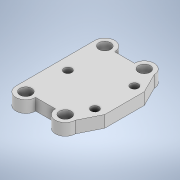
# Autodesk Inventor part: Camera_Mount_DFK33GP006
Saved by Autodesk Inventor 2021 (Build 250183000, 183)
## iProperties
Created: 2022-02-02
Part Number: Camera_Mount_DFK33GP006
Material: Generic
Document SubType Name: Modeling
Designer: Jorian Brusind
Density: 1 g/cm^3
Appearance: Default
Author: Jorian Brusind
Autodesk Inventor part; units mm, degrees
ref_plane "YZ Plane" through (0, 0, 0) normal (1, 0, 0) x (0, 1, 0)
ref_plane "XZ Plane" through (0, 0, 0) normal (0, 1, 0) x (-1, 0, 0)
ref_plane "XY Plane" through (0, 0, 0) normal (0, 0, 1) x (1, 0, 0)
sketch "Sketch1" plane through (0, 0, 0) normal (0, 1, 0) x (-1, 0, 0)
  line L0 (0, 0) -> (40, 0)
  line L1 (40, 0) -> (40, -50)
  line L2 (40, -50) -> (0, -50)
  line L3 (0, -50) -> (0, 0)
  line L4 (0, -25) -> (5, -25)
  line L5 (5, -25) -> (28.7, -25)
  line L6 (5, -25) -> (5, -15)
  line L7 (5, -25) -> (5, -35)
  circle A0 centre (5, -15) radius 2
  circle A1 centre (5, -35) radius 2
  circle A2 centre (28.7, -25) radius 2
  line L8 (40, 0) -> (30, 0)
  line L9 (30, 0) -> (30, -5)
  circle A3 centre (30, -5) radius 3
  circle A4 centre (30, -45) radius 3
  circle A5 centre (10, -5) radius 3
  circle A6 centre (10, -45) radius 3
  circle A7 centre (30, -5) radius 5
  circle A8 centre (10, -5) radius 5
  circle A9 centre (30, -45) radius 5
  circle A10 centre (10, -45) radius 5
  line L10 (0, -15) -> (5, -15)
  line L11 (5, -35) -> (0, -35)
  line L12 (10, -5) -> (5, -5)
  line L13 (5, -5) -> (0, -15)
  line L14 (5, -23) -> (28.7, -23)
  line L15 (28.7, -23) -> (28.7, -27)
  line L16 (28.7, -27) -> (5, -27)
  line L17 (5, -27) -> (5, -23)
  line L18 (5, -23) -> (28.7, -27) construction
  line L19 (28.7, -23) -> (5, -27) construction
  line L20 (25, -5) -> (25, -23)
  line L21 (25, -27) -> (25, -45)
  line L22 (30, -5) -> (35, -5)
  line L23 (35, -5) -> (35, -45)
  line L24 (15, -5) -> (15, -23)
  line L25 (15, -45) -> (15, -27)
  line L26 (0, -35) -> (5, -45)
  line L27 (25, -45) -> (15, -45)
  line L28 (25, -5) -> (15, -5)
  point P0 (10, 0)
  point P1 (30, -40)
  point P2 (10, -40)
  point P3 (16.85, -25)
  point P4 (33, -5)
  point P5 (30, -2)
  dimension "d0" = 40
  dimension "d1" = 50
  dimension "d2" = 5
  dimension "d3" = 23.7
  dimension "d4" = 10
  dimension "d5" = 10
  dimension "d6" = 4
  dimension "d7" = 4
  dimension "d8" = 4
  dimension "d9" = 10
  dimension "d10" = 5
  dimension "d11" = 6
  dimension "d14" = 40
  dimension "d17" = 20
  dimension "d22" = 20
  dimension "d25" = 40
  dimension "d28" = 23.7
  dimension "d29" = 4
  dimension "d30" = 18
  dimension "d31" = 18
  dimension "d32" = 18
  dimension "d33" = 18
  dimension "d34" = 10
  constraints: 58 end point, 12 point on circle, 11 centre point, 8 point on line, 7 horizontal, 7 perpendicular, 6 parallel, 5 coincident, 4 midpoint, 3 vertical, 2 tangent, 15 other
  measures "d0" distance of L1.end L2.end
  measures "d1" distance of L0.end L1.end
  measures "d2" distance of L4.start L4.end
  measures "d3" distance of L4.end L5.end
  measures "d4" distance of L4.end L6.end
  measures "d5" distance of L4.end L7.end
  measures "d6" diameter of A0
  measures "d7" diameter of A1
  measures "d8" diameter of A2
  measures "d9" distance of L0.end L8.end
  measures "d10" distance of L8.end L9.end
  measures "d11" diameter of A3
  measures "d14" distance of A3.centre A4.centre
  measures "d17" distance of A3.centre A5.centre
  measures "d22" distance of L22.start L12.start
  measures "d25" distance of L22.start A9.centre
  measures "d28" distance of L15.end L16.end
  measures "d29" distance of L14.end L15.end
  measures "d30" distance of L20.start L20.end
  measures "d31" distance of L21.start L21.end
  measures "d32" distance of L24.start L24.end
  measures "d33" distance of L25.start L25.end
  measures "d34" vertical distance of L11.end L26.end
extrude "Extrusion1" add sketch "Sketch1" along normal blind 6 contours A7 L22 A3 L9 | L9 A3 L22 A7 | A8 | L23 A9 L21 L16 A2 L14 L20 A7 | L20 L14 L24 L28 | L24 L14 L6 A0 L10 L13 A8 | A9 | L14 A2 L5 L6 | L10 A0 L6 L4 L3 | L27 L25 L16 L21 | A10 | L4 L7 A1 L11 L3 | L16 L7 L5 A2 | A10 L26 L11 A1 L7 L16 L25
body "Solid1"
